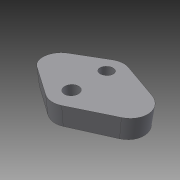
# Autodesk Inventor part: z_axis_top_cap
Saved by Autodesk Inventor 2014 (Build 180170000, 170)
## iProperties
Created: 2013-12-09
Part Number: z_axis_top_cap
Material: Generic
Document SubType Name: Modeling
Designer: buben
Density: 1 g/cm^3
Appearance: Default
Author: buben
Subject: Laser Cutted
Autodesk Inventor part; units mm, degrees
ref_plane "YZ Plane" through (0, 0, 0) normal (1, 0, 0) x (0, 1, 0)
ref_plane "XZ Plane" through (0, 0, 0) normal (0, 1, 0) x (-1, 0, 0)
ref_plane "XY Plane" through (0, 0, 0) normal (0, 0, 1) x (1, 0, 0)
sketch "Sketch1" plane through (0, 0, 0) normal (0, 0, 1) x (1, 0, 0)
  circle A0 centre (0, 0) radius 4 construction
  circle A1 centre (23, 0) radius 2.5 construction
  arc A2 (-2.7754, 5.3195) -> (-2.7754, -5.3195) centre (0, 0) ccw
  arc A3 (25.7754, -5.3195) -> (25.7754, 5.3195) centre (23, 0) ccw
  circle A4 centre (11.5, 6) radius 2.25
  line L0 (0, 0) -> (23, 0) construction
  circle A5 centre (11.5, -6) radius 2.25
  line L1 (11.5, 6) -> (11.5, -6) construction
  circle A6 centre (11.5, 6) radius 4.5 construction
  arc A7 (14.2754, 11.3195) -> (8.7246, 11.3195) centre (11.5, 6) ccw
  arc A8 (8.7246, -11.3195) -> (14.2754, -11.3195) centre (11.5, -6) ccw
  line L2 (8.7246, 11.3195) -> (-2.7754, 5.3195)
  line L3 (14.2754, 11.3195) -> (25.7754, 5.3195)
  line L4 (8.7246, -11.3195) -> (-2.7754, -5.3195)
  line L5 (25.7754, -5.3195) -> (14.2754, -11.3195)
  point P0 (11.5, 0)
  dimension "d0" = 8
  dimension "d1" = 5
  dimension "d2" = 23
  dimension "d3" = 12
  dimension "d4" = 4.5
  dimension "d5" = 9
  dimension "d6" = 12
  dimension "d7" = 12
  constraints: 12 end point, 9 centre point, 8 point on circle, 8 tangent, 6 coincident, 3 equal radius, 2 midpoint, 1 horizontal, 1 horizontal alignment, 1 perpendicular, 1 vertical alignment
  measures "d0" diameter of A0
  measures "d1" diameter of A1
  measures "d2" distance of A1.centre point (0, 0)
  measures "d3" diameter of A2
  measures "d4" diameter of A4
  measures "d5" diameter of A6
  measures "d6" diameter of A7
  measures "d7" distance of L1.start L1.end
extrude "Extrusion1" add sketch "Sketch1" along normal blind 6
body "Solid1"
